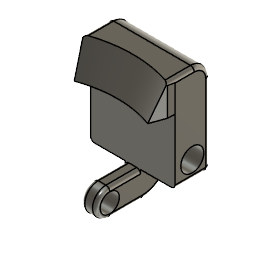
fixture2 (Autodesk Fusion 360 design; units mm, degrees)
part number: 2026-07-27-19-13-52-002
Autodesk Fusion 360 part; units mm, degrees
note: some values were not read from the file. Set by a fixed rule: which sketch regions a step uses.
sketch "스케치1" plane through (0, 0, 0) normal (1, 0, 0) x (0, 1, 0)
  line L0 (-6, 12) -> (-85, 12)
  line L1 (-6, 7) -> (-6, 12)
  line L2 (34.5, 8) -> (32, 8)
  line L3 (-85, 12) -> (-85, 7)
  line L4 (35, 0) -> (35, -12)
  line L5 (0, 0) -> (-2.4947, 0)
  line L6 (-85, 7) -> (-6, 7)
  line L7 (35, -12) -> (37, -12)
  line L8 (-14, 12) -> (-23, 12)
  line L9 (28, -2) -> (28.9985, -2)
  line L10 (0, 0) -> (28, 0)
  line L11 (-2.4947, 0) -> (-1.4931, -2)
  line L12 (-6, 7) -> (-2.4947, 0)
  line L13 (30, 0) -> (28.9985, -2)
  line L14 (0, -2) -> (0, 0)
  circle A0 centre (-15, -7) radius 4
  line L15 (35, -12) -> (-85, -12)
  line L16 (-6, 12) -> (-85, 12)
  circle A1 centre (-15, -7) radius 10
  line L17 (0, -2) -> (-1.4931, -2)
  line L18 (-6, 7) -> (1.8286, 7) construction
  line L19 (28, -2) -> (0, -2)
  line L20 (37, 6) -> (37, 8)
  line L21 (32, 8) -> (34.5, 8)
  line L22 (0, 0) -> (28, 0)
  line L23 (28, 0) -> (28, -2)
  line L24 (-85, -12) -> (-85, 12)
  line L25 (37, -12) -> (37, 8)
  line L26 (28, 0) -> (30, 0)
  line L27 (35, 0) -> (35, -12)
  line L28 (30, 0) -> (36.7103, 0) construction
  line L29 (35, -8) -> (35, -4)
  line L30 (0, 0) -> (-6, 12)
  line L31 (30, 4) -> (28, 0)
  line L32 (14, 0) -> (14, 8.2971)
  line L33 (30, 0) -> (30, 4)
  line L34 (30, 4) -> (30, 8)
  line L35 (30, 4) -> (28, 4)
  line L36 (28, 4) -> (30, 8)
  line L37 (30, 8) -> (34.5, 8)
  line L38 (30, 4) -> (30, -4.5)
  line L39 (34.5, 8) -> (34.5, -4.5)
  line L40 (34.5, -4.5) -> (30, -4.5)
  line L41 (30, -4.5) -> (34.5, -4.5)
  line L42 (34.5, -4.5) -> (34.5, 0)
  line L43 (34.5, 0) -> (30, 0)
  line L44 (30, 0) -> (30, -4.5)
  circle A2 centre (32.25, -2.25) radius 1.5
  line L45 (30, -4.5) -> (34.5, -4.5)
  line L46 (30.5, -6) -> (30.5, -4.5)
  line L47 (34, -6) -> (34, -4.5)
  line L48 (33.9918, -5.8306) -> (34, -5.8333)
  line L49 (30.5082, -5.8306) -> (30.5, -5.8333)
  line L50 (30.5, -4.5) -> (34, -4.5)
  line L51 (34, -4.5) -> (34, -8)
  line L52 (34, -8) -> (30.5, -8)
  line L53 (30.5, -8) -> (30.5, -4.5)
  line L54 (30.5, -8) -> (26, -8)
  line L55 (26, -8) -> (26, -4.5)
  line L56 (26, -4.5) -> (30.5, -4.5)
  line L57 (30.5, -4.5) -> (30.5, -8)
  circle A3 centre (26, -6.25) radius 1.75
  circle A4 centre (26, -6.25) radius 1.25
  point P0 (-15, -7)
  point P1 (-2, 4)
  dimension "d1" = 28
  dimension "d4" = 120
  dimension "d5" = 8
  dimension "d6" = 20
  dimension "d7" = 5
  dimension "d9" = 2
  dimension "d11" = 2
  dimension "d12" = 63.4
  dimension "d14" = 4
  dimension "d15" = 4
  dimension "d16" = 2
  dimension "d17" = 3
  dimension "d18" = 4.5
  dimension "d40" = 3.5
  dimension "d41" = 4.5
  dimension "d42" = 3.5
  dimension "d43" = 2.5
  constraint coincident L5.start L10.start
  constraint horizontal L22
  constraint perpendicular L4 L21
  constraint horizontal L15
  constraint perpendicular L15 L24
  constraint vertical L29
  constraint coincident L29.end L4
  constraint horizontal L8
  constraint coincident L8.start L0
  constraint coincident P0 A0.centre
  constraint perpendicular L3 L16
  constraint parallel L6 L16
  constraint parallel L1 L3
  constraint perpendicular L16 L24
  constraint perpendicular L7 L27
  constraint parallel L25 L27
  constraint perpendicular L15 L27
  constraint parallel L22 L26
  constraint horizontal L28
  constraint perpendicular L10 L23
  constraint parallel L10 L19
  constraint parallel L14 L23
  constraint perpendicular L9 L23
  constraint perpendicular L5 L14
  constraint horizontal L18
  constraint parallel L11 L12
  constraint perpendicular L14 L17
  constraint vertical L32
  constraint midpoint L10 L32.start
  constraint perpendicular L26 L33
  constraint coincident L31.start L33.end
  constraint parallel L33 L34
  constraint perpendicular L34 L35
  constraint perpendicular L34 L37
  constraint perpendicular L35 L38
  constraint perpendicular L21 L39
  constraint perpendicular L38 L40
  constraint horizontal L41
  constraint vertical L42
  constraint horizontal L43
  constraint vertical L44
  constraint coincident L28 L42.end
  constraint coincident L39 L42.end
  constraint coincident L28 L4.start
  constraint horizontal L45
  constraint coincident L45 L46.end
  constraint perpendicular L45 L46
  constraint coincident L45 L47.end
  constraint perpendicular L45 L47
  constraint coincident L46 L49.end
  constraint coincident L47 L48.end
  constraint horizontal L50
  constraint vertical L51
  constraint horizontal L52
  constraint vertical L53
  constraint horizontal L54
  constraint vertical L55
  constraint horizontal L56
  constraint vertical L57
  constraint midpoint L55 A3.centre
  constraint coincident L54.end A3
  constraint concentric A3 A4
  measures "d1" distance of L5.start L10.end
  measures "d4" distance of L15.end L4.end
  measures "d5" diameter of A0
  measures "d6" diameter of A1
  measures "d7" distance of L0.start L1.start
  measures "d9" distance of L20.end L20.start
  measures "d11" distance of L5.start L14.start
  measures "d12" angle of L12 L18
  measures "d14" distance of L13.start L31.start
  measures "d15" distance of L31.start L34.end
  measures "d16" distance of L31.start L35.end
  measures "d17" diameter of A2
  measures "d18" distance of L38.end L39.end
  measures "d40" distance of L46.end L52.end
  measures "d41" distance of L52.end L54.end
  measures "d42" distance of L52.end L46.end
  measures "d43" diameter of A4
extrude "돌출1" add sketch "스케치1" along normal blind 5.5 contours L38 L39 L40 L41 L42 L43 L44 L45 L50 L56 | L2 L21 L33 L34 L37 L38 L39 L43 makes body 1
extrude "돌출2" add sketch "스케치1" against normal blind 5.5 contours L38 L39 L40 L41 L42 L43 L44 L45 L50 L56 | L2 L21 L33 L34 L37 L38 L39 L43 bodies 1
revolve "회전1" add sketch "스케치1" angle 20 about axis through (0, 14, 0) along (0, 0, 1) second angle 20 separate body contours L34 L35 L36 makes body 2
sketch "스케치2" plane through (0, 30, 0) normal (0, -1, 0) x (1, 0, 0)
  line L0 (-5.5, -4.5) -> (5.5, -4.5)
  line L1 (5.5, -4.5) -> (5.5, 8)
  line L2 (5.5, 8) -> (-5.5, 8)
  line L3 (-5.5, 8) -> (-5.5, -4.5)
  line L4 (-5.5, 8) -> (5.5, 8)
  line L5 (5.5, 8) -> (5.5, 4)
  line L6 (5.5, 4) -> (-5.5, 4)
  line L7 (-5.5, 4) -> (-5.5, 8)
  constraint horizontal L4
  constraint vertical L5
  constraint horizontal L6
  constraint vertical L7
  constraint coincident L1 L5.end
  constraint coincident L2.end L3.start
loft "로프트1" add profiles "스케치2" section 1 contours L1 L2 L3 L4 L5 L6 L7 section 2 face at (-0.3723, 29.9957, 5.3333) on bodies 2 bodies 1 2
extrude "돌출7" add sketch "스케치1" along normal blind 1 contours L40 L41 L45 L46 L53 L54 L56 L57 A3 | L40 L41 L45 L46 L47 L50 L51 L52 L53 L57 | L55 A3 A4 | L55 A3 A4 bodies 1
extrude "돌출8" add sketch "스케치1" against normal blind 1 contours L40 L41 L45 L46 L53 L54 L56 L57 A3 | L40 L41 L45 L46 L47 L50 L51 L52 L53 L57 | L55 A3 A4 | L55 A3 A4 bodies 1
fillet "필렛3" radius 2 1 edges at (0, 34.5, 8) on bodies 1
fillet "필렛4" radius 0.5 9 edges at (-5.5, 31.25, 8) (-5.5, 33.9142, 7.4142) (-5.5, 34.5, 0.75) (-5.5, 32.25, -4.5) (0, 34.5, -4.5) (5.5, 34.5, 0.75) (5.5, 33.9142, 7.4142) (5.5, 31.25, 8) (5.5, 32.25, -4.5) on bodies 1
fillet "필렛5" radius 3.75 1 edges at (0, 34, -8) on bodies 1
fillet "필렛6" radius 0.5 8 edges at (1, 28, -4.5) (1, 24.25, -6.25) (1, 28.1292, -8) (1, 32.8201, -6.9886) (-1, 32.8201, -6.9886) (-1, 28.1292, -8) (-1, 24.25, -6.25) (-1, 28, -4.5) on bodies 1
